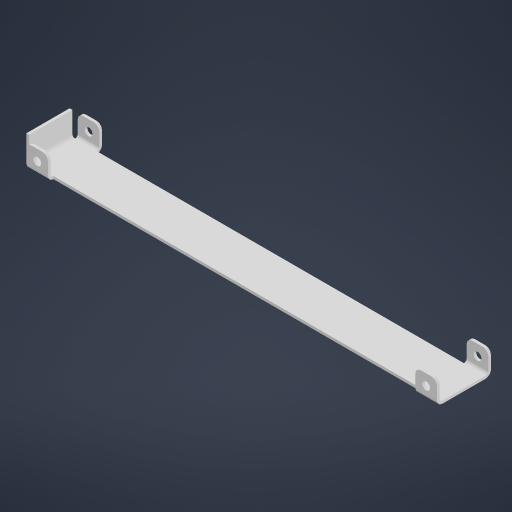
# Autodesk Inventor part: wingcovers
Saved by Autodesk Inventor 2024 (Build 280153000, 153)
## iProperties
Created: 2023-09-02
Part Number: wingcovers
Material: Generic
Document SubType Name: Sheet Metal
Designer: reima
Density: 1 g/cm^3
Sheet Metal Rule: Default
Appearance: Default
Flat Pattern Width: 5.3975 cm
Flat Pattern Length: 25.7175 cm
Flat Pattern Area: 138.81 cm^2
Sheet Metal Width: 2.125 in
Sheet Metal Length: 10.125 in
Sheet Metal Area: 21.516 in^2
Author: reima
Autodesk Inventor part; units mm, degrees
ref_plane "YZ Plane" through (0, 0, 0) normal (1, 0, 0) x (0, 1, 0)
ref_plane "XZ Plane" through (0, 0, 0) normal (0, 1, 0) x (-1, 0, 0)
ref_plane "XY Plane" through (0, 0, 0) normal (0, 0, 1) x (1, 0, 0)
sketch "Sketch1" plane through (0, 0, 0) normal (0, 1, 0) x (-1, 0, 0)
  line L0 (0, 25.4) -> (-257.175, 25.4)
  line L1 (-257.175, 25.4) -> (-257.175, 0)
  line L2 (-257.175, 0) -> (0, 0)
  line L3 (0, 0) -> (0, 25.4)
  circle A0 centre (-250.825, 19.05) radius 2.3368
  circle A1 centre (-250.825, 6.35) radius 2.3368
  circle A2 centre (-22.225, 19.05) radius 2.3368
  circle A3 centre (-22.225, 6.35) radius 2.3368
  line L4 (-257.175, 25.4) -> (-244.475, 25.4)
  line L5 (-244.475, 25.4) -> (-244.475, 36.5125)
  line L6 (-247.65, 39.6875) -> (-254, 39.6875)
  line L7 (-257.175, 36.5125) -> (-257.175, 25.4)
  circle A4 centre (-250.825, 33.3375) radius 2.3368
  line L8 (-257.175, 12.7) -> (0, 12.7) construction
  line L9 (-257.175, 0) -> (-244.475, 0)
  line L10 (-244.475, 0) -> (-244.475, -11.1125)
  line L11 (-247.65, -14.2875) -> (-254, -14.2875)
  line L12 (-257.175, -11.1125) -> (-257.175, 0)
  circle A5 centre (-250.825, -7.9375) radius 2.3368
  line L13 (-136.525, 25.4) -> (-136.525, 0) construction
  line L14 (-28.575, 25.4) -> (-28.575, 36.5125)
  line L15 (-25.4, 39.6875) -> (-19.05, 39.6875)
  line L16 (-15.875, 36.5125) -> (-15.875, 25.4)
  circle A6 centre (-22.225, 33.3375) radius 2.3368
  circle A7 centre (-22.225, -7.9375) radius 2.3368
  line L17 (-25.4, -14.2875) -> (-19.05, -14.2875)
  line L18 (-15.875, -11.1125) -> (-15.875, 0)
  line L19 (-28.575, 0) -> (-28.575, -11.1125)
  arc A8 (-15.875, 36.5125) -> (-19.05, 39.6875) centre (-19.05, 36.5125) ccw
  arc A9 (-25.4, 39.6875) -> (-28.575, 36.5125) centre (-25.4, 36.5125) ccw
  arc A10 (-28.575, -11.1125) -> (-25.4, -14.2875) centre (-25.4, -11.1125) ccw
  arc A11 (-19.05, -14.2875) -> (-15.875, -11.1125) centre (-19.05, -11.1125) ccw
  arc A12 (-247.65, -14.2875) -> (-244.475, -11.1125) centre (-247.65, -11.1125) ccw
  arc A13 (-257.175, -11.1125) -> (-254, -14.2875) centre (-254, -11.1125) ccw
  arc A14 (-254, 39.6875) -> (-257.175, 36.5125) centre (-254, 36.5125) ccw
  arc A15 (-244.475, 36.5125) -> (-247.65, 39.6875) centre (-247.65, 36.5125) ccw
  point P0 (0, 0)
  point P1 (-244.475, 39.6875)
  point P2 (-257.175, 39.6875)
  point P3 (-250.825, 39.6875)
  point P4 (-244.475, -14.2875)
  point P5 (-257.175, -14.2875)
  point P6 (-250.825, -14.2875)
  point P7 (-28.575, 39.6875)
  point P8 (-15.875, 39.6875)
  point P9 (-28.575, -14.2875)
  point P10 (-15.875, -14.2875)
  point P11 (-244.475, 0)
  point P12 (-28.575, 0)
  point P13 (-15.875, 0)
  point P14 (-15.875, 25.4)
  point P15 (-28.575, 25.4)
  point P16 (-244.475, 25.4)
  dimension "d0" = 257.175
  dimension "d1" = 25.4
  dimension "d2" = 4.6736
  dimension "d3" = 4.6736
  dimension "d4" = 6.35
  dimension "d5" = 6.35
  dimension "d6" = 12.7
  dimension "d7" = 6.35
  dimension "d8" = 4.6736
  dimension "d9" = 4.6736
  dimension "d10" = 12.7
  dimension "d11" = 6.35
  dimension "d12" = 6.35
  dimension "d13" = 228.6
  dimension "d14" = 0
  dimension "d15" = 0
  dimension "d16" = 12.7
  dimension "d17" = 14.2875
  dimension "d18" = 4.6736
  dimension "d19" = 6.35
  dimension "d20" = 114.3
  dimension "d21" = 3.175
  measures "d0" distance of L2.end L1.end
  measures "d1" distance of L0.end L1.end
  measures "d2" diameter of A0
  measures "d3" diameter of A1
  measures "d4" distance from line of L1 A0.centre
  measures "d5" distance from line of L1 A1.centre
  measures "d6" distance of A1.centre A0.centre
  measures "d7" distance from line of L0 A0.centre
  measures "d8" diameter of A2
  measures "d9" diameter of A3
  measures "d10" distance of A3.centre A2.centre
  measures "d11" distance from line of L2 A3.centre
  measures "d12" distance from line of L0 A2.centre
  measures "d13" distance of A0.centre A2.centre
  measures "d14" distance from line of point (0, 0) L2
  measures "d15" distance from line of point (0, 0) L3
  measures "d16" distance of point (-257.175, 39.687) point (-244.475, 39.687)
  measures "d17" distance of point (-244.475, 39.687) L4.end
  measures "d18" diameter of A4
  measures "d19" distance of point (-250.825, 39.687) A4.centre
  measures "d20" distance from line of A1.centre L13
  measures "d21" radius of A8
extrude "Plate1" add sketch "Sketch1" along normal blind 1.5875 contours L3 L2 L1 L0 | L0 L14 A9 L15 A8 L16 | L18 A11 L17 A10 L19 L2 | L0 L7 A14 L6 A15 L5 | L10 A12 L11 A13 L12 L2 | A0 | A1 | A2 | A3
sketch "Sketch2" plane through (0, 1.5875, 0) normal (0, 1, 0) x (1, 0, 0)
  line L0 (15.875, -25.4) -> (0, -25.4) projected
  line L1 (15.875, -25.4) -> (28.6122, -25.4)
  line L2 (15.875, 0) -> (15.875, 11.1125) projected
  line L3 (244.475, 0) -> (28.575, 0) projected
  line L4 (15.875, 0) -> (28.575, 0)
  line L5 (244.475, 0) -> (257.7147, 0)
  line L6 (28.575, -25.4) -> (244.475, -25.4) projected
  line L7 (244.475, -25.4) -> (257.175, -25.4)
  line L8 (257.175, -36.5125) -> (257.175, 11.1125) projected
  line L9 (15.875, -25.4) -> (15.875, 0)
  point P0 (0, 0)
  constraints: 10 end point, 4 horizontal, 1 perpendicular, 1 point on line
fold "Fold1" angle 90 bend radius 1.5875 thickness 1.5875 k factor 0.44 line from (15.875, 1.5875, 25.4) to (15.875, 1.5875, 0) line at bend start moving side (-1, 0, 0) folds toward (0, 1, 0)
fold "Fold2" angle 90 bend radius 1.5875 thickness 1.5875 k factor 0.44 line from (244.475, 1.5875, 25.4) to (257.175, 1.5875, 25.4) line at bend start moving side (0, 0, 1) folds toward (0, 1, 0)
fold "Fold3" angle 90 bend radius 1.5875 thickness 1.5875 k factor 0.44 line from (15.875, 1.5875, 0) to (28.575, 1.5875, 0) line at bend start moving side (0, 0, -1) folds toward (0, 1, 0)
sketch "Sketch3" plane through (0, 1.5875, 0) normal (0, 1, 0) x (1, 0, 0)
  line L0 (15.875, -25.4) -> (28.575, -25.4)
  line L1 (244.475, 0) -> (257.175, 0)
  line L2 (257.175, -25.4) -> (257.175, 11.1125) projected
  point P0 (0, 0)
  constraints: 4 end point, 2 horizontal, 1 point on line
fold "Fold4" angle 90 bend radius 1.5875 thickness 1.5875 k factor 0.44 line from (244.475, 1.5875, 0) to (257.175, 1.5875, 0) line at bend start moving side (0, 0, -1) folds toward (0, 1, 0)
fold "Fold5" angle 90 bend radius 1.5875 thickness 1.5875 k factor 0.44 line from (15.875, 1.5875, 25.4) to (28.575, 1.5875, 25.4) line at bend start moving side (0, 0, 1) folds toward (0, 1, 0)
unfold all bends "Unfold1" k factor 0.44 fixed face at (172.5083, 1.5875, 16.9333)
refold all bends "Refold1"
equation "\"d22\" = Thickness"
equation "\"d23\" = BendReliefWidth"
equation "\"d25\" = MinimumRemnant"
equation "\"d26\" = TransitionRadius"
equation "\"d29\" = BendReliefWidth"
equation "\"d31\" = MinimumRemnant"
equation "\"d32\" = TransitionRadius"
equation "\"d35\" = BendReliefWidth"
equation "\"d37\" = MinimumRemnant"
equation "\"d38\" = TransitionRadius"
equation "\"d41\" = BendReliefWidth"
equation "\"d43\" = MinimumRemnant"
equation "\"d44\" = TransitionRadius"
equation "\"d47\" = BendReliefWidth"
equation "\"d49\" = MinimumRemnant"
equation "\"d50\" = TransitionRadius"
equation "\"BendRadius\" = Thickness"
equation "\"BendReliefWidth\" = Thickness"
equation "\"BendReliefDepth\" = 0.5 * Thickness"
equation "\"CornerReliefSize\" = 4 * Thickness"
equation "\"MinimumRemnant\" = 2 * Thickness"
equation "\"TransitionRadius\" = BendRadius"
equation "\"JacobiRadiusSize\" = BendRadius"
equation "\"GapSize\" = Thickness"
equation "\"Thickness\" = 1.5875"
body "Solid1"
